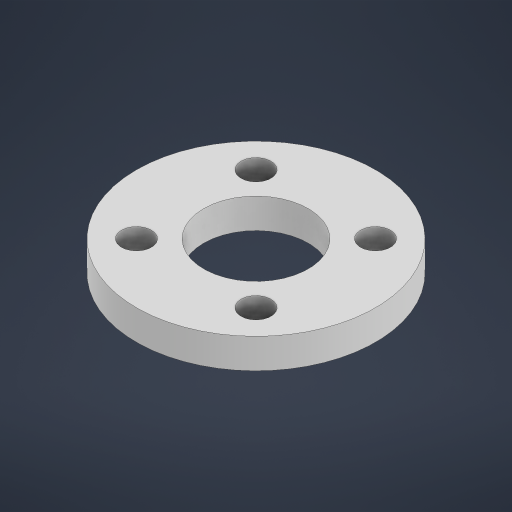
# Autodesk Inventor part: MotorPulleySpacer
Saved by Autodesk Inventor 2024 (Build 280153000, 153)
## iProperties
Created: 2023-10-28
Part Number: MotorPulleySpacer
Material: Generic
Document SubType Name: Modeling
Designer: avsar
Density: 1 g/cm^3
Appearance: Default
Author: avsar
Autodesk Inventor part; units mm, degrees
ref_plane "YZ Plane" through (0, 0, 0) normal (1, 0, 0) x (0, 1, 0)
ref_plane "XZ Plane" through (0, 0, 0) normal (0, 1, 0) x (-1, 0, 0)
ref_plane "XY Plane" through (0, 0, 0) normal (0, 0, 1) x (1, 0, 0)
sketch "Sketch1" plane through (0, 0, 0) normal (0, 1, 0) x (-1, 0, 0)
  circle A0 centre (0, 0) radius 7
  circle A1 centre (0, 0) radius 16
  circle A2 centre (8, 8) radius 2
  circle A3 centre (-8, 8) radius 2
  circle A4 centre (-8, -8) radius 2
  circle A5 centre (8, -8) radius 2
  dimension "d0" = 14
  dimension "d1" = 32
  dimension "d4" = 4
  dimension "d5" = 8
  dimension "d6" = 8
  dimension "d9" = 360
  constraints: 6 centre point, 2 coincident, 9 other
  measures "d0" diameter of A0
  measures "d1" diameter of A1
  measures "d4" diameter of A2
  measures "d5" horizontal distance of point (0, 0) A2.centre
  measures "d6" horizontal distance of point (0, 0) A2.centre
extrude "Extrusion1" add sketch "Sketch1" along normal blind 4
body "Solid1"
